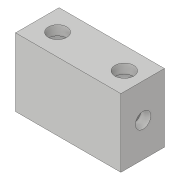
# Autodesk Inventor part: body_of_the_bot
Saved by Autodesk Inventor 2019 (Build 230136000, 136)
## iProperties
Created: 2019-10-14
Part Number: body_of_the_bot
Material: Generic
Document SubType Name: Modeling
Designer: Lenovo
Density: 1 g/cm^3
Appearance: Default
Author: Lenovo
Autodesk Inventor part; units mm, degrees
ref_plane "YZ Plane" through (0, 0, 0) normal (1, 0, 0) x (0, 1, 0)
ref_plane "XZ Plane" through (0, 0, 0) normal (0, 1, 0) x (-1, 0, 0)
ref_plane "XY Plane" through (0, 0, 0) normal (0, 0, 1) x (1, 0, 0)
sketch "Sketch1" plane through (0, 0, 0) normal (0, 0, 1) x (1, 0, 0)
  line L0 (10.8783, -7.0389) -> (-10.8783, -7.0389)
  line L1 (-10.8783, -7.0389) -> (-10.8783, 7.0389)
  line L2 (-10.8783, 7.0389) -> (10.8783, 7.0389)
  line L3 (10.8783, 7.0389) -> (10.8783, -7.0389)
  line L4 (10.8783, -7.0389) -> (-10.8783, 7.0389) construction
  line L5 (-10.8783, -7.0389) -> (10.8783, 7.0389) construction
  point P0 (0, 0)
  constraints: 12 end point, 2 midpoint, 2 parallel, 1 horizontal, 1 perpendicular
extrude "Extrusion1" add sketch "Sketch1" along normal blind 9
sketch "Sketch2" plane through (-10.8783, 7.0389, 0) normal (0, 1, 0) x (1, 0, 0)
  circle A0 centre (4.2234, -4.5433) radius 1.9026
  circle A1 centre (18.0126, -4.5433) radius 1.9371
  point P0 (10.8783, 0)
  constraints: 2 centre point
extrude "Extrusion2" cut sketch "Sketch2" against normal blind 2
sketch "Sketch3" plane through (10.8783, -7.0389, 0) normal (1, 0, 0) x (0, 0, -1)
  circle A0 centre (-4.4153, 7.0389) radius 1.5998
  point P0 (0, 7.0389)
  constraints: 1 centre point
extrude "Extrusion3" cut sketch "Sketch3" against normal blind 2
sketch "Sketch4" plane through (-10.8783, -7.0389, 0) normal (0, -1, 0) x (1, 0, 0)
  circle A0 centre (18.0126, 4.5433) radius 1.9371 projected
  circle A1 centre (18.0126, 4.5433) radius 1.9371
  circle A2 centre (3.4358, 4.4153) radius 2.0338
  point P0 (10.8783, 0)
  constraints: 2 centre point, 1 coincident
extrude "Extrusion4" cut sketch "Sketch4" against normal blind 2
body "Solid1"
